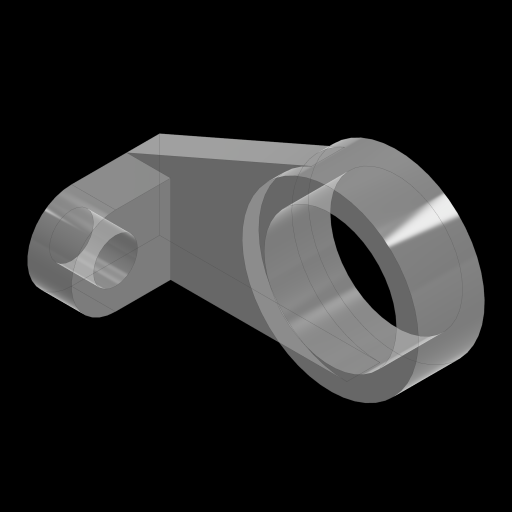
# Autodesk Inventor part: ANS7-4-BK
Saved by Autodesk Inventor 2024 (Build 280153000, 153)
## iProperties
Created: 2023-10-27
Part Number: ANS7-4-BK
Material: PET Plastic
Document SubType Name: Modeling
Designer: bennk
Density: 1.541 g/cm^3
Appearance: Polycarbonate - Clear
Mass: 463.986 g
Surface Area: 517.244 cm^2
Volume: 301.094 cm^3
Author: bennk
Autodesk Inventor part; units mm, degrees
ref_plane "YZ Plane" through (0, 0, 0) normal (1, 0, 0) x (0, 1, 0)
ref_plane "XZ Plane" through (0, 0, 0) normal (0, 1, 0) x (-1, 0, 0)
ref_plane "XY Plane" through (0, 0, 0) normal (0, 0, 1) x (1, 0, 0)
sketch "Sketch1" plane through (0, 0, 0) normal (0, 0, 1) x (1, 0, 0)
  circle A0 centre (0, 0) radius 50.8
  line L0 (0, -50.8) -> (-127, -50.8)
  line L1 (-127, -50.8) -> (-127, 0)
  line L2 (-127, 0) -> (-20.32, 46.559)
  dimension "d0" = 127
  dimension "d1" = 101.6
  dimension "d2" = 50.8
  constraints: 6 end point, 2 point on circle, 2 tangent, 1 centre point, 1 coincident, 1 horizontal, 1 perpendicular
  measures "d0" distance of L0.start L0.end
  measures "d1" diameter of A0
  measures "d2" distance of L0.end L1.end
extrude "MAIN BODY" add sketch "Sketch1" along normal mid plane 19.05
sketch "Sketch2" plane through (0, 0, 0) normal (0, 0, 1) x (1, 0, 0)
  arc A0 (0, -50.8) -> (-20.32, 46.559) centre (0, 0) ccw projected
  circle A1 centre (0, 0) radius 50.8
  point P0 (0, -50.8)
  dimension "d5" = 101.6
  constraints: 1 centre point, 1 coincident
  measures "d5" diameter of A1
extrude "MAIN BODY LIP" add sketch "Sketch2" along normal mid plane 38.1
sketch "Sketch3" plane through (0, 0, 9.525) normal (0, 0, 1) x (1, 0, 0)
  line L0 (-127, -50.8) -> (0, -50.8) projected
  line L1 (-127, -50.8) -> (-101.6, -50.8)
  line L2 (-101.6, -50.8) -> (-101.6, 0)
  line L3 (-101.6, 0) -> (-127, 0)
  line L4 (-127, 0) -> (-127, -50.8)
  point P0 (0, 0)
  point P1 (-101.6, -25.4)
  dimension "d8" = 25.4
  dimension "d9" = 50.8
  constraints: 8 end point, 2 parallel, 1 horizontal, 1 midpoint, 1 perpendicular
  measures "d8" distance from line of point (-101.6, -25.4) L4
  measures "d9" distance between parallel lines of L0 L3
extrude "SIDE EXT" add sketch "Sketch3" along normal blind 31.75
sketch "Sketch4" plane through (-101.6, -50.8, 9.525) normal (1, 0, 0) x (0, 0, -1)
  line L0 (-31.75, 0) -> (-31.75, 50.8) projected
  circle A0 centre (-31.75, 25.4) radius 25.4
  point P0 (9.525, 50.8)
  constraints: 1 midpoint, 3 other
extrude "SIDE EXT CURVE" add sketch "Sketch4" against normal blind 25.4 contours A0 L0 picked at (-40.1549, 26.4205)
sketch "Sketch5" plane through (-101.6, -50.8, 9.525) normal (1, 0, 0) x (0, 0, -1)
  arc A0 (-31.75, 50.8) -> (-31.75, 0) centre (-31.75, 25.4) ccw projected
  point P0 (9.525, 50.8)
  constraints: 1 coincident
hole "SIDE EXT HOLE" at (-101.6, -25.4, 41.275) direction (-1, 0, 0) diameter 25.4 end through all
sketch "Sketch6" plane through (0, 0, 19.05) normal (0, 0, 1) x (1, 0, 0)
  circle A0 centre (0, 0) radius 50.8 projected
  constraints: 1 coincident
hole "MAIN BODY HOLE" at (0, 0, 19.05) direction (0, 0, -1) diameter 76.2 end through all
body "Solid1"
